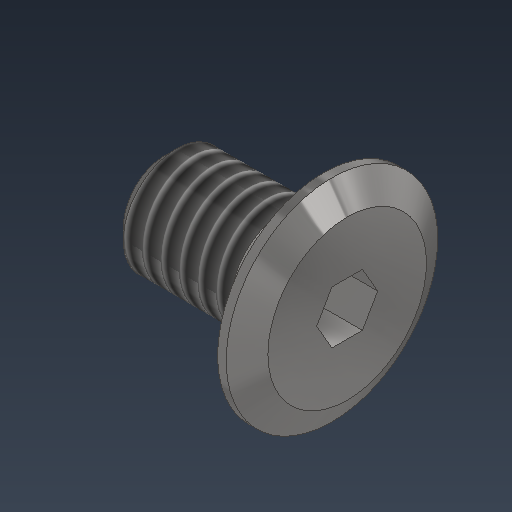
# Autodesk Inventor part: CBSTSR4-6
Saved by Autodesk Inventor 2021 (Build 250183000, 183)
## iProperties
Category: PARTsolutions
Company: MISUMI
Part Number: CBSTSR4-6
Material: 鋼、炭素鋼
Catalog Web Link: www.cadenas.de
Description: CBSTSR,CBSTBR,CBSTNR-Ultra Low Head Cap Screws - Hex Sockets
Vendor: MISUMI
Document SubType Name: Modeling
Designer: partserver
Manufacturer: MISUMI
Mass: 0.791206 g
Surface Area: 2.02285 cm^2
Volume: 0.100791 cm^3
Density: 7.85 g/cm^3
Appearance: 半つや出し
PSOL_IDENT_0: {$CADENAS_DATA\23d-libs\misumi\metric\27_screws_nuts\cbstsr.prj},181 {VTYP=3D},{NB=CBSTSR4-6},{LINA=
PSOL_IDENT_1: CBSTSR4-6},{NN=CBSTSR,CBSTBR,CBSTNR},{DATE=03.06.2021 03:35:26},{GEOMDATE=04.03.2020 04:03:33},{VERS
PSOL_IDENT_2: ION=},{LINEID=20},{WBVAR=MAT,ST,L},{WBNUMERIC=L}  {NB=CBSTSR4-6},{LINA=CBSTSR4-6},{KT=DUMMY},{PN=CBS
PSOL_IDENT_3: TSR4-6},{TYPE=CBSTSR},{MAT=SUS304},{HARD=-},{ST=-},{STALG='-','-'},{STPN=},{M=4.0},{L=6},{LALG=5,6,8
PSOL_IDENT_4: ,10,12,14,16,18,20,25},{LS=5,6,8,10,12,14,16,18,20,25},{LNB=5,6,8,10,12,16},{P=0.70},{MP=M4x0.7},{A=
PSOL_IDENT_5: 8},{B=2.0},{E=0.9},{TT=2.5},{EE=1.5},{RR=0.20},{AA=1}
NB: CBSTSR4-6
NN: CBSTSR,CBSTBR,CBSTNR
NT: Ultra Low Head Cap Screws - Hex Sockets
NBSYN: $PN.
LINA: CBSTSR4-6
CATALOG: Misumi
PN: CBSTSR4-6
TYPE: CBSTSR
MAT: 304 Stainless Steel
HARD: -
ST: -
M: 4
L: 6
LS: 5,6,8,10,12,14,16,18,20,25
LNB: 5,6,8,10,12,16
MP: M4x0.7
A: 8
B: 2
E: 0.9
TT: 2.5
EE: 1.5
RR: 0.2
SUPPLIER: MISUMI
ARTICLENO: CBSTSR4-6
BOMINFO: CBSTSR4-6
CREATOR: CADENAS GmbH
在庫数: 0.0
購入先: ミスミ
Title: CBSTSR4-6
Author: Cadenas PARTsolutions
Comments: Ultra Low Head Cap Screws - Hex Sockets
Autodesk Inventor part; units mm, degrees
ref_plane "YZ Plane" through (0, 0, 0) normal (1, 0, 0) x (0, 1, 0)
ref_plane "XZ Plane" through (0, 0, 0) normal (0, 1, 0) x (-1, 0, 0)
ref_plane "XY Plane" through (0, 0, 0) normal (0, 0, 1) x (1, 0, 0)
sketch "Sketch_1" plane through (0, 0, 0) normal (0, 0, 1) x (1, 0, 0)
  line L0 (6, 0) -> (-0.9, 0)
  line L1 (-0.9, 0) -> (-0.9, 3)
  line L2 (-0.9, 3) -> (-0.3226, 4)
  line L3 (-0.3226, 4) -> (0, 4)
  line L4 (0, 4) -> (0, 1.9852)
  arc A0 (0, 1.9852) -> (0.2, 1.7853) centre (0.2, 1.9853) ccw
  line L5 (0.2, 1.7853) -> (0.8, 1.7853)
  line L6 (0.8, 1.7853) -> (1.5, 2)
  line L7 (1.5, 2) -> (5.5705, 2)
  line L8 (5.5705, 2) -> (6, 1.5705)
  line L9 (6, 1.5705) -> (6, 0)
  line L10 (6, 0) -> (-0.9, 0)
  constraints: 22 end point, 2 point on circle, 1 centre point
revolve "Revolution1" add sketch "Sketch_1" angle 360 about axis through (6, 0, 0) along (1, 0, 0)
thread "Thread1" size "M4x0.7" class "6g" standard "ISO Metric profile" full length
sketch "Sketch2" plane through (-0.9, 0, 0) normal (-1, 0, 0) x (0, 0, 1)
  point P0 (0, 0)
hole "Hole1" at (-0.9, 0, 0) direction (1, 0, 0) diameter 2 depth 2.5 tip angle 120
sketch "Sketch_3" plane through (-0.9, 0, 0) normal (1, 0, 0) x (0, 0, -1)
  line L0 (-1, -0.5774) -> (0, -1.1547)
  line L1 (0, -1.1547) -> (1, -0.5774)
  line L2 (1, -0.5774) -> (1, 0.5774)
  line L3 (1, 0.5774) -> (0, 1.1547)
  line L4 (0, 1.1547) -> (-1, 0.5774)
  line L5 (-1, 0.5774) -> (-1, -0.5774)
  constraints: 12 end point
extrude "Extrusion1" cut sketch "Sketch_3" along normal blind 2.5
body "Solid1"
